Sleeping Room  Cabinet (Autodesk Fusion 360 design; units mm, degrees)
Autodesk Fusion 360 part; units mm, degrees
sketch "Sketch1" plane through (0, 0, 0) normal (0, 1, 0) x (1, 0, 0)
  line L0 (0, 0) -> (120, 0)
  line L1 (120, 0) -> (120, -241.9)
  line L2 (0, 0) -> (0, -64.6)
  line L3 (0, -64.6) -> (120, -241.9)
  line L4 (120, 0) -> (123, 0)
  line L5 (123, 0) -> (123, -241.9)
  line L6 (123, -241.9) -> (120, -241.9)
  line L7 (120, -241.9) -> (120, 0)
  line L8 (-3, 3) -> (223, 3)
  line L9 (223, 3) -> (223, -244.9)
  line L10 (223, -244.9) -> (-3, -244.9)
  line L11 (-3, -244.9) -> (-3, 3)
  line L12 (-3, 3) -> (223, 3)
  line L13 (223, 3) -> (223, 0)
  line L14 (223, 0) -> (-3, 0)
  line L15 (-3, 0) -> (-3, 3)
  line L16 (-3, -244.9) -> (223, -244.9)
  line L17 (223, -244.9) -> (223, -241.9)
  line L18 (223, -241.9) -> (-3, -241.9)
  line L19 (-3, -241.9) -> (-3, -244.9)
  dimension "d1" = 120
  dimension "d2" = 241.9
  dimension "d3" = 64.6
  dimension "d4" = 3
  dimension "d7" = 3
  dimension "d8" = 3
  dimension "d9" = 3
  dimension "d10" = 241.9
  dimension "d11" = 100
  dimension "d12" = 3
  constraint coincident L0.start L2.start
  constraint horizontal L0
  constraint perpendicular L0 L1
  constraint perpendicular L0 L2
  constraint horizontal L4
  constraint vertical L5
  constraint horizontal L6
  constraint vertical L7
  constraint horizontal L8
  constraint vertical L9
  constraint horizontal L10
  constraint vertical L11
  constraint horizontal L12
  constraint vertical L13
  constraint horizontal L14
  constraint vertical L15
  constraint coincident L9 L13.end
  constraint horizontal L16
  constraint vertical L17
  constraint horizontal L18
  constraint vertical L19
  measures "d1" distance of L0.start L0.end
  measures "d2" distance of L0.end L1.end
  measures "d3" distance of L0.start L2.end
  measures "d4" distance of L0.end L4.end
  measures "d7" distance of L0 L8
  measures "d8" distance of L2 L11
  measures "d9" distance of L6 L10
  measures "d10" distance of L4.end L5.end
  measures "d11" distance of L5 L9
  measures "d12" distance of L10.end L18.end
extrude "Extrude1" add sketch "Sketch1" along normal blind 400 contours L0 L4 L8 L9 L11 L12 L13 L14 L15 | L2 L3 L11 L14 L18 | L6 L9 L10 L11 L16 L17 L18 L19
